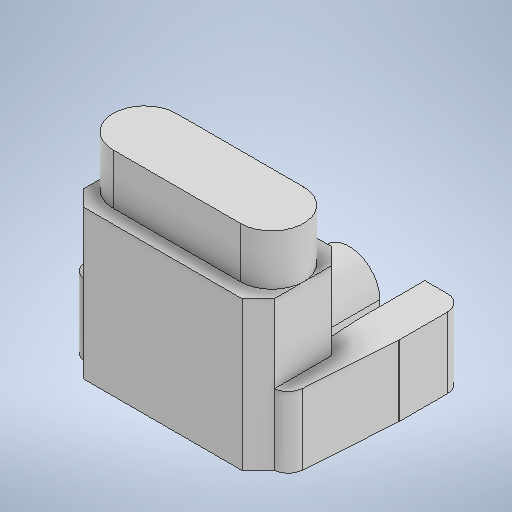
# Autodesk Inventor part: SecondarySecure
Saved by Autodesk Inventor 2027 (Build 310192060, 192F)
## iProperties
Created: 2026-07-07
Part Number: SecondarySecure
Material: Generic
Document SubType Name: Modeling
Designer: 13129
Density: 1 g/cm^3
Appearance: Default
Author: 13129
Autodesk Inventor part; units mm, degrees
ref_plane "YZ Plane" through (0, 0, 0) normal (1, 0, 0) x (0, 1, 0)
ref_plane "XZ Plane" through (0, 0, 0) normal (0, 1, 0) x (-1, 0, 0)
ref_plane "XY Plane" through (0, 0, 0) normal (0, 0, 1) x (1, 0, 0)
sketch "Sketch1" plane through (0, 0, 0) normal (0, 0, 1) x (1, 0, 0)
  circle A0 centre (0, 0) radius 6.1
  line L0 (-6.1, 0) -> (-6.1, -6.1)
  line L1 (-6.1, -6.1) -> (6.1, -6.1)
  line L2 (6.1, -6.1) -> (6.1, 0)
  dimension "d0" = 12.2
  constraints: 6 end point, 3 tangent, 2 point on circle, 2 vertical, 1 centre point, 1 coincident, 1 perpendicular
  measures "d0" diameter of A0
extrude "Extrusion1" add sketch "Sketch1" along normal blind 19.05
sketch "Sketch2" plane through (0, 0, 19.05) normal (0, 0, 1) x (1, 0, 0)
  arc A0 (6.1, 0) -> (-6.1, 0) centre (0, 0) ccw construction
  line L0 (-6.1, 0) -> (-6.1, -6.1) construction
  line L1 (6.1, -6.1) -> (6.1, 0) construction
  line L2 (-6.1, -6.1) -> (-6.1, 6.1)
  line L3 (-6.1, 6.1) -> (6.1, 6.1)
  line L4 (6.1, 6.1) -> (6.1, -6.1)
  line L5 (-6.1, -6.1) -> (6.1, -6.1)
  constraints: 8 end point, 1 collinear, 1 horizontal, 1 perpendicular, 1 point on line, 1 tangent
extrude "Extrusion2" add sketch "Sketch2" along normal blind 17.78
sketch "Sketch3" plane through (0, 6.1, 19.05) normal (0, 1, 0) x (1, 0, 0)
  line L0 (0, 0) -> (-6.1, 0) construction
  line L1 (-12.6, -8.79) -> (12.6, -8.79) construction
  line L2 (-12.6, -15.04) -> (12.6, -15.04)
  line L3 (12.6, -2.54) -> (-12.6, -2.54)
  arc A0 (-12.6, -2.54) -> (-12.6, -15.04) centre (-12.6, -8.79) ccw
  arc A1 (12.6, -15.04) -> (12.6, -2.54) centre (12.6, -8.79) ccw
  point P0 (0, 19.05)
  point P1 (0, -8.79)
  point P2 (0, -2.54)
  dimension "d5" = 2.54
  dimension "d6" = 25.2
  dimension "d7" = 12.5
  constraints: 8 end point, 4 point on circle, 4 tangent, 2 centre point, 2 midpoint, 1 horizontal, 1 parallel, 1 vertical alignment
  measures "d5" distance between parallel lines of L0 L3
  measures "d6" distance of L2.start L2.end
  measures "d7" distance between parallel lines of L3 L2
extrude "Extrusion3" add sketch "Sketch3" along normal blind 27.25
sketch "Sketch4" plane through (0, 6.1, 19.05) normal (0, -1, 0) x (1, 0, 0)
  arc A0 (12.6, 2.54) -> (12.6, 15.04) centre (12.6, 8.79) ccw construction
  line L0 (-18.85, 0) -> (18.85, 0)
  line L1 (18.85, 0) -> (18.85, 17.78)
  line L2 (18.85, 17.78) -> (-18.85, 17.78)
  line L3 (-18.85, 17.78) -> (-18.85, 0)
  arc A1 (-12.6, 15.04) -> (-12.6, 2.54) centre (-12.6, 8.79) ccw construction
  line L4 (-6.1, 17.78) -> (6.1, 17.78) construction
  point P0 (0, -19.05)
  point P1 (-18.85, 8.79)
  point P2 (18.85, 8.79)
  point P3 (0, 17.78)
  point P4 (0, 0)
  constraints: 8 end point, 2 horizontal alignment, 2 parallel, 2 point on circle, 2 vertical alignment, 1 horizontal, 1 midpoint, 1 perpendicular
extrude "Extrusion4" add sketch "Sketch4" against normal blind 17.25
sketch "Sketch5" plane through (0, 6.1, 19.05) normal (0, -1, 0) x (1, 0, 0)
  line L0 (-18.85, 0) -> (-6.1, 0) construction
  line L1 (18.85, 17.78) -> (-18.85, 17.78)
  line L2 (-18.85, 17.78) -> (-18.85, 0)
  line L3 (-18.85, 0) -> (18.85, 0)
  line L4 (18.85, 0) -> (18.85, 17.78)
  point P0 (0, -19.05)
  constraints: 8 end point, 2 parallel, 1 horizontal, 1 perpendicular
extrude "Extrusion5" add sketch "Sketch5" along normal up to surface (12.2 mm away)
chamfer "Chamfer1" distance 3.175 angle 45 4 edges at (18.85, 8.625, 19.05) (18.85, 8.625, 36.83) (-18.85, 8.625, 19.05) (-18.85, 8.625, 36.83)
sketch "Sketch6" plane through (-6.1, -6.1, 0) normal (0, -1, 0) x (1, 0, 0)
  line L0 (0, 0) -> (12.2, 0) construction
  line L1 (24.95, 33.655) -> (24.95, 22.225) construction
  line L2 (-9.575, 36.83) -> (21.775, 36.83) construction
  line L3 (21.3, 12.9) -> (21.3, 0.2)
  line L4 (24.95, 27.84) -> (24.95, 22.225) construction
  line L5 (24.95, 22.225) -> (21.775, 22.225)
  line L6 (21.775, 22.225) -> (21.3, 12.9)
  line L7 (24.95, 22.225) -> (24.95, 33.655)
  line L8 (24.95, 33.655) -> (27.49, 33.655)
  line L9 (27.49, 33.655) -> (28.92, 12.9)
  line L10 (28.92, 12.9) -> (28.92, 0.2)
  line L11 (28.92, 0.2) -> (21.3, 0.2)
  line L12 (6.1, 0) -> (6.1, 36.83)
  line L13 (-12.75, 22.225) -> (-9.575, 19.05) construction
  line L14 (-12.75, 33.655) -> (-12.75, 22.225) construction
  line L15 (-9.1, 12.9) -> (-9.1, 0.2)
  line L16 (-12.75, 27.84) -> (-12.75, 22.225) construction
  line L17 (-12.75, 22.225) -> (-9.575, 22.225)
  line L18 (-9.575, 22.225) -> (-9.1, 12.9)
  line L19 (-12.75, 22.225) -> (-12.75, 33.655)
  line L20 (-12.75, 33.655) -> (-15.29, 33.655)
  line L21 (-15.29, 33.655) -> (-16.72, 12.9)
  line L22 (-16.72, 12.9) -> (-16.72, 0.2)
  line L23 (-16.72, 0.2) -> (-9.1, 0.2)
  point P0 (6.1, 0)
  dimension "d17" = 15.2
  dimension "d19" = 0.2
  dimension "d21" = 7.62
  dimension "d23" = 12.7
  dimension "d28" = 2.54
  dimension "d29" = 3.175
  constraints: 40 end point, 7 symmetric about line, 2 horizontal, 2 midpoint, 2 perpendicular, 1 collinear, 1 horizontal alignment, 1 vertical
  measures "d17" distance from line of L12.start L3
  measures "d19" distance between parallel lines of L11 L0
  measures "d21" distance of L9.end L3.start
  measures "d23" distance of L3.start L3.end
  measures "d28" distance of L1.start L8.end
  measures "d29" distance of L1.end L5.end
extrude "Extrusion6" add sketch "Sketch6" against normal blind 14
fillet "Fillet1" radius 3.175 6 edges at (21.39, 0.9, 33.655) (-21.39, 0.9, 33.655) (-22.82, 0.9, 0.2) (-22.82, 0.9, 12.9) (22.82, 0.9, 0.2) (22.82, 0.9, 12.9)
body "Solid1"
